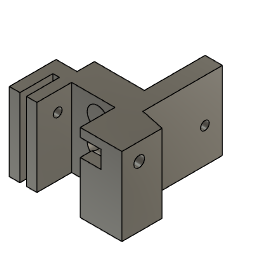
LeviDrzacZaALUProfilKojiDrziALUProfilSaGolmanom v4 (Autodesk Fusion 360 design; units mm, degrees)
Autodesk Fusion 360 part; units mm, degrees
note: some values were not read from the file. Set by a fixed rule: which sketch regions a step uses.
sketch "Sketch4" plane through (0, 0, 0) normal (0, 0, 1) x (1, 0, 0)
  line L0 (10, 0) -> (17, 0)
  line L1 (17, 0) -> (17, 20)
  line L2 (17, 20) -> (35, 20)
  line L3 (42, 27) -> (10, 27)
  line L4 (35, 20) -> (35, 0)
  line L5 (35, 0) -> (42, 0)
  line L6 (42, 0) -> (220, 0)
  line L7 (220, 0) -> (220, 27)
  line L8 (220, 27) -> (42, 27)
  line L9 (10, 27) -> (0, 27)
  line L10 (0, 0) -> (6.2, 0)
  line L11 (6.2, 0) -> (6.2, 19)
  line L12 (6.2, 19) -> (10, 19)
  line L13 (10, 19) -> (10, 0)
  line L14 (0.0791, 27) -> (0, 27)
  line L15 (0, 27) -> (0, 0)
  line L16 (0, 0) -> (0.0791, 0)
  line L17 (0.0791, 0) -> (0.0791, 27)
  dimension "d6" = 7
  dimension "d10" = 178
  dimension "d11" = 27
  dimension "d12" = 3.8
  constraint horizontal L0
  constraint vertical L1
  constraint horizontal L2
  constraint horizontal L3
  constraint vertical L4
  constraint horizontal L5
  constraint horizontal L6
  constraint vertical L7
  constraint horizontal L8
  constraint horizontal L9
  constraint horizontal L10
  constraint vertical L11
  constraint horizontal L12
  constraint vertical L13
  constraint horizontal L14
  constraint vertical L15
  constraint horizontal L16
  constraint vertical L17
  constraint coincident L10.start L15.end
  constraint coincident L9 L14.start
  constraint coincident L15 L10.start
  measures "d6" distance of L0.start L0.end
  measures "d10" distance of L5.end L6.end
  measures "d11" distance of L5.end L3.start
  measures "d12" distance of L0.start L10.end
extrude "Extrude1" add sketch "Sketch4" along normal blind 17 contours L0 L1 L2 L3 L4 L5 L6 L7 L8 L9 L10 L11 L12 L13 L17 makes body 1
sketch "Sketch5" plane through (0, 0, 0) normal (1, 0, 0) x (0, 1, 0)
  circle A0 centre (12, 9) radius 2.5
  dimension "d16" = 5
  measures "d16" diameter of A0
extrude "Extrude2" cut sketch "Sketch5" along normal blind 30 bodies 1
sketch "Sketch6" plane through (0, 0, 17) normal (0, 0, 1) x (-1, 0, 0)
  line L0 (-6.2, 0) -> (-6.2, -19)
  line L1 (-6.2, -19) -> (-10, -19)
  line L2 (-10, -19) -> (-10, 0)
  line L3 (-10, 0) -> (-17, 0)
  line L4 (-17, 0) -> (-17, -20)
  line L5 (-17, -20) -> (-35, -20)
  line L6 (-35, -20) -> (-35, 0)
  line L7 (-35, 0) -> (-220, 0)
  line L8 (-220, 0) -> (-220, -27)
  line L9 (-220, -27) -> (-0.0791, -27)
  line L10 (-0.0791, -27) -> (-0.0791, 0)
  line L11 (-0.0791, 0) -> (-6.2, 0)
  line L12 (-220, -27) -> (-42, -27)
  line L13 (-42, -27) -> (-42, -20)
  line L14 (-42, -20) -> (-220, -20)
  line L15 (-220, -20) -> (-220, -27)
  dimension "d19" = 178
  dimension "d20" = 7
  constraint horizontal L12
  constraint vertical L13
  constraint horizontal L14
  constraint vertical L15
  constraint coincident L8.end L9.start
  measures "d19" distance of L8.end L12.end
  measures "d20" distance of L8.end L14.end
extrude "Extrude3" cut sketch "Sketch6" against normal blind 60 contours L8 L9 L12 L13 L14 L15 bodies 1
sketch "Sketch7" plane through (0, 0, 17) normal (0, 0, 1) x (-1, 0, 0)
  line L0 (-42, -20) -> (-42, -27)
  line L1 (-42, -27) -> (-0.0791, -27)
  line L2 (-0.0791, -27) -> (-0.0791, 0)
  line L3 (-0.0791, 0) -> (-6.2, 0)
  line L4 (-6.2, 0) -> (-6.2, -19)
  line L5 (-6.2, -19) -> (-10, -19)
  line L6 (-10, -19) -> (-10, 0)
  line L7 (-10, 0) -> (-17, 0)
  line L8 (-17, 0) -> (-17, -20)
  line L9 (-17, -20) -> (-35, -20)
  line L10 (-35, -20) -> (-35, 0)
  line L11 (-35, 0) -> (-220, 0)
  line L12 (-220, 0) -> (-220, -20)
  line L13 (-220, -20) -> (-42, -20)
  line L14 (-42, -27) -> (-75, -20)
  constraint coincident L0.end L1.start
  constraint coincident L13 L14.end
extrude "Extrude4" add sketch "Sketch7" against normal blind 17 contours L0 L13 L14 bodies 1
sketch "Sketch8" plane through (0, 0, 17) normal (0, 0, 1) x (-1, 0, 0)
  line L0 (-42, -27) -> (-0.0791, -27)
  line L1 (-0.0791, -27) -> (-0.0791, 0)
  line L2 (-0.0791, 0) -> (-6.2, 0)
  line L3 (-6.2, 0) -> (-6.2, -19)
  line L4 (-6.2, -19) -> (-10, -19)
  line L5 (-10, -19) -> (-10, 0)
  line L6 (-10, 0) -> (-17, 0)
  line L7 (-17, 0) -> (-17, -20)
  line L8 (-17, -20) -> (-35, -20)
  line L9 (-35, -20) -> (-35, 0)
  line L10 (-35, 0) -> (-220, 0)
  line L11 (-220, 0) -> (-220, -20)
  line L12 (-220, -20) -> (-75, -20)
  line L13 (-75, -20) -> (-42, -27)
  line L14 (-17, -37) -> (-37, -37)
  line L15 (-17, -37) -> (-37, -37)
  line L16 (-37, -37) -> (-37, -85.9394)
  line L17 (-37, -85.9394) -> (-47, -85.9394)
  line L18 (-47, -85.9394) -> (-47, -25.9394)
  line L19 (-17, -37) -> (-17, -87)
  line L20 (-17, -87) -> (-7.161, -87)
  line L21 (-7.161, -87) -> (-7.161, -27)
  dimension "d26" = 20
  dimension "d27" = 10
  dimension "d28" = 60
  dimension "d29" = 60
  constraint perpendicular L14 L16
  constraint perpendicular L16 L17
  constraint coincident L13 L18.end
  constraint perpendicular L17 L18
  constraint perpendicular L14 L19
  constraint perpendicular L19 L20
  constraint coincident L0 L21.end
  constraint perpendicular L0 L21
  measures "d26" distance of L14.start L14.end
  measures "d27" distance of L16.end L17.end
  measures "d28" distance of L20.end L21.end
  measures "d29" distance of L17.end L18.end
extrude "Extrude5" add sketch "Sketch8" along normal blind 3 bodies 1
extrude "Extrude6" add 1 faces at (43.6667, 49.6263, 17) along direction (0, 0, -1) blind 17 on bodies 1 bodies 1
sketch "Sketch9" plane through (0, 20, 0) normal (0, -1, 0) x (1, 0, 0)
  line L0 (17, 0) -> (35, 0)
  line L1 (35, 0) -> (35, 20)
  line L2 (35, 20) -> (17, 20)
  line L3 (17, 20) -> (17, 0)
extrude "Extrude7" cut 1 faces at (35, 6.6667, 13.3333) along direction (1, 0, 0) blind 1 on bodies 1 bodies 1
extrude "Extrude8" cut 1 faces at (17, 3.176, 9.7909) along direction (-1, 0, 0) blind 1 on bodies 1 bodies 1
sketch "Sketch10" plane through (0, 20, 0) normal (0, -1, 0) x (1, 0, 0)
  arc A0 (26, 13.1) -> (22.9, 10) centre (26, 10) ccw
  circle A1 centre (26, 10) radius 3.1
  dimension "d40" = 6.2
  dimension "d41" = 6.2
  constraint concentric A0 A1
  measures "d40" diameter of A0
  measures "d41" diameter of A1
extrude "Extrude9" cut sketch "Sketch10" against normal blind 20 bodies 1
sketch "Sketch11" plane through (0, 20, 0) normal (0, -1, 0) x (1, 0, 0)
  circle A0 centre (26, 10) radius 6
  dimension "d44" = 12
  measures "d44" diameter of A0
extrude "Extrude10" cut sketch "Sketch11" against normal blind 5 bodies 1
sketch "Sketch12" plane through (47, 0, 0) normal (1, 0, 0) x (0, 1, 0)
  line L0 (85.9394, 0) -> (85.9394, 20)
  line L1 (85.9394, 20) -> (25.9394, 20)
  line L2 (25.9394, 20) -> (25.9394, 0)
  line L3 (25.9394, 0) -> (85.9394, 0)
  circle A0 centre (60, 10) radius 2.5
  dimension "d47" = 5
  measures "d47" diameter of A0
extrude "Extrude11" cut sketch "Sketch12" against normal blind 50 contours A0 bodies 1
sketch "Sketch13" plane through (0, 0, 20) normal (0, 0, 1) x (-1, 0, 0)
  line L0 (-16, -20) -> (-36, -20)
  line L1 (-36, -20) -> (-36, 0)
  line L2 (-36, 0) -> (-220, 0)
  line L3 (-220, 0) -> (-220, -20)
  line L4 (-220, -20) -> (-75, -20)
  line L5 (-75, -20) -> (-47, -25.9394)
  line L6 (-47, -25.9394) -> (-47, -85.9394)
  line L7 (-47, -85.9394) -> (-37, -85.9394)
  line L8 (-37, -85.9394) -> (-37, -37)
  line L9 (-37, -37) -> (-17, -37)
  line L10 (-17, -37) -> (-17, -87)
  line L11 (-17, -87) -> (-7.161, -87)
  line L12 (-7.161, -87) -> (-7.161, -27)
  line L13 (-7.161, -27) -> (-0.0791, -27)
  line L14 (-0.0791, -27) -> (-0.0791, 0)
  line L15 (-0.0791, 0) -> (-6.2, 0)
  line L16 (-6.2, 0) -> (-6.2, -19)
  line L17 (-6.2, -19) -> (-10, -19)
  line L18 (-10, -19) -> (-10, 0)
  line L19 (-10, 0) -> (-16, 0)
  line L20 (-16, 0) -> (-16, -20)
extrude "Extrude12" add 1 faces at (43.6667, 85.9394, 6.6667) along direction (0, 1, 0) blind 1.061 on bodies 1 bodies 1
sketch "Sketch14" plane through (0, 0, 20) normal (0, 0, 1) x (-1, 0, 0)
sketch "Sketch15" plane through (0, 37, 0) normal (0, 1, 0) x (-1, 0, 0)
  circle A0 centre (-26, 10) radius 3.1
  line L0 (-17, 0) -> (-17, 20)
  line L1 (-17, 20) -> (-37, 20)
  line L2 (-37, 20) -> (-37, 0)
  line L3 (-37, 0) -> (-17, 0)
  line L4 (-37, 10) -> (-27, 10)
  dimension "d52" = 10
  constraint midpoint L2 L4.start
  constraint perpendicular L2 L4
  measures "d52" distance of L4.start L4.end
extrude "Extrude13" add sketch "Sketch15" against normal blind 12 contours A0 bodies 1
sketch "Sketch16" plane through (0, 0, 20) normal (0, 0, 1) x (-1, 0, 0)
extrude "Extrude14" cut 1 faces at (17, 78.8333, 10) along direction (-1, 0, 0) blind 1 on bodies 1 bodies 1
sketch "Sketch17" plane through (0, 0, 20) normal (0, 0, 1) x (-1, 0, 0)
extrude "Extrude15" add 1 faces at (37, 78.8336, 10) along direction (-1, 0, 0) blind 1 on bodies 1 bodies 1
extrude "Extrude16" cut 1 faces at (47, 36.4596, 10) along direction (-1, 0, 0) blind 1 on bodies 1 bodies 1
sketch "Sketch18" plane through (0, 37, 0) normal (0, 1, 0) x (-1, 0, 0)
  line L0 (-36, 20) -> (-36, 0)
  line L1 (-36, 0) -> (-16, 0)
  line L2 (-16, 0) -> (-16, 20)
  line L3 (-16, 20) -> (-36, 20)
  circle A0 centre (-26, 10) radius 3.1
  dimension "d61" = 6.2
  measures "d61" diameter of A0
extrude "Extrude17" cut sketch "Sketch18" against normal blind 29 contours A0 bodies 1
sketch "Sketch19" plane through (0, 0, 20) normal (0, 0, 1) x (-1, 0, 0)
sketch "Sketch20" plane through (0, 0, 20) normal (0, 0, 1) x (-1, 0, 0)
  line L0 (-220, 0) -> (-60, 0)
  line L1 (-60, 0) -> (-60, -35)
  line L2 (-60, -35) -> (-237.965, -35)
  line L3 (-237.965, -35) -> (-237.965, 0)
  line L4 (-237.965, 0) -> (-220, 0)
  dimension "d64" = 160
  constraint horizontal L0
  constraint perpendicular L0 L1
  constraint perpendicular L1 L2
  constraint perpendicular L2 L3
  constraint perpendicular L3 L4
  measures "d64" distance of L0.start L0.end
extrude "Extrude18" cut sketch "Sketch20" against normal blind 40 bodies 1
sketch "Sketch21" plane through (60, 0, 0) normal (1, 0, 0) x (0, 1, 0)
  line L0 (23.1818, 0) -> (23.1818, 20)
  line L1 (23.1818, 20) -> (0, 20)
  line L2 (0, 20) -> (0, 0)
  line L3 (0, 0) -> (23.1818, 0)
  line L4 (0, 10) -> (10, 10)
  circle A0 centre (10, 10) radius 3.1
  dimension "d67" = 6.2
  constraint midpoint L2 L4.start
  constraint perpendicular L2 L4
  constraint coincident L4.end A0.centre
  measures "d67" diameter of A0
extrude "Extrude19" cut sketch "Sketch21" against normal blind 31 contours A0 bodies 1
sketch "Sketch22" plane through (36, 0, 0) normal (-1, 0, 0) x (0, -1, 0)
  circle A0 centre (-10, 10) radius 3.1
  line L0 (-20, 0) -> (0, 0)
  line L1 (0, 0) -> (0, 20)
  line L2 (0, 20) -> (-20, 20)
  line L3 (-20, 20) -> (-20, 0)
  circle A1 centre (-10, 10) radius 6
  dimension "d70" = 12
  constraint concentric A0 A1
  measures "d70" diameter of A1
extrude "Extrude20" cut sketch "Sketch22" against normal blind 6 contours A1 bodies 1
sketch "Sketch23" plane through (0, 0, 0) normal (0, -1, 0) x (1, 0, 0)
  line L0 (60, 0) -> (60, 20)
  line L1 (60, 20) -> (36, 20)
  line L2 (36, 20) -> (36, 0)
  line L3 (36, 0) -> (60, 0)
  line L4 (36, 15.0296) -> (48, 15.0296)
  line L5 (48, 15.0296) -> (48, 5)
  line L6 (48, 5) -> (36, 5)
  line L7 (36, 5) -> (36, 15.0296)
  dimension "d73" = 24
  dimension "d74" = 12
  constraint horizontal L4
  constraint vertical L5
  constraint horizontal L6
  constraint vertical L7
  constraint coincident L2 L4.start
  measures "d73" distance of L0.end L1.end
  measures "d74" distance of L4.start L4.end
extrude "Extrude21" cut sketch "Sketch23" against normal blind 10 contours L2 L4 L5 L6 L7 bodies 1
sketch "Sketch24" plane through (0, 0, 20) normal (0, 0, 1) x (-1, 0, 0)
sketch "Sketch25" plane through (0, 0, 0) normal (0, 0, -1) x (1, 0, 0)
  line L0 (60, -23.1818) -> (60, 0)
  line L1 (60, 0) -> (36, 0)
  line L2 (36, 0) -> (36, -20)
  line L3 (36, -20) -> (16, -20)
  line L4 (16, -20) -> (16, 0)
  line L5 (16, 0) -> (10, 0)
  line L6 (10, 0) -> (10, -19)
  line L7 (10, -19) -> (6.2, -19)
  line L8 (6.2, -19) -> (6.2, 0)
  line L9 (6.2, 0) -> (0.0791, 0)
  line L10 (0.0791, 0) -> (0.0791, -27)
  line L11 (0.0791, -27) -> (7.161, -27)
  line L12 (7.161, -27) -> (7.161, -87)
  line L13 (7.161, -87) -> (16, -87)
  line L14 (16, -87) -> (16, -37)
  line L15 (16, -37) -> (36, -37)
  line L16 (36, -37) -> (36, -87.0004)
  line L17 (36, -87.0004) -> (46, -87.0004)
  line L18 (46, -87.0004) -> (46, -25.9394)
  line L19 (46, -25.9394) -> (47, -25.9394)
  line L20 (47, -25.9394) -> (60, -23.1818)
  line L21 (46, -25.9394) -> (46, 0)
  line L22 (7.161, -27) -> (7.161, -19)
  constraint coincident L18.end L19.start
  constraint coincident L1 L21.end
  constraint perpendicular L1 L21
  constraint coincident L11.end L12.start
  constraint coincident L7 L22.end
  constraint perpendicular L7 L22
extrude "Extrude22" add sketch "Sketch25" along normal blind 15 contours L1 L2 L3 L4 L5 L6 L7 L12 L13 L14 L15 L16 L17 L18 L21 L22 bodies 1
sketch "Sketch26" plane through (0, 37, 0) normal (0, 1, 0) x (-1, 0, 0)
  circle A0 centre (-26, 10) radius 3.1
  line L0 (-36, 20) -> (-36, -15)
  line L1 (-36, -15) -> (-16, -15)
  line L2 (-16, -15) -> (-16, 20)
  line L3 (-16, 20) -> (-36, 20)
  circle A1 centre (-26, 10) radius 3.1
  constraint concentric A0 A1
extrude "Extrude23" add sketch "Sketch26" against normal blind 17 contours A0 A1 bodies 1
sketch "Sketch27" plane through (26, 20, 10) normal (0, -1, 0) x (1, 0, 0)
  circle A0 centre (0, 0) radius 5.984
  constraint coincident A0.centre origin
extrude "Extrude24" cut sketch "Sketch27" against normal blind 6 bodies 1
delete_face "DeleteFace1" 1 faces at (24.7178, 26, 11.1628) on bodies 1
sketch "Sketch28" plane through (26, 20, 10) normal (0, -1, 0) x (1, 0, 0)
sketch "Sketch29" plane through (0, 37, 0) normal (0, 1, 0) x (-1, 0, 0)
  line L0 (-36, 20) -> (-36, -15)
  line L1 (-36, -15) -> (-16, -15)
  line L2 (-16, -15) -> (-16, 20)
  line L3 (-16, 20) -> (-36, 20)
  circle A0 centre (-26, 10) radius 5.984
  circle A1 centre (-26, 10) radius 5.984
  constraint concentric A0 A1
extrude "Extrude25" add sketch "Sketch29" against normal blind 18 contours A0 A1 bodies 1
extrude "Extrude26" cut 1 faces at (24.2692, 19, 9.9802) along direction (0, 1, 0) blind 1 on bodies 1 bodies 1
sketch "Sketch30" plane through (46, 0, 0) normal (1, 0, 0) x (0, 1, 0)
  circle A0 centre (60, 10) radius 2.5
  line L0 (87.0004, 20) -> (25.9394, 20)
  line L1 (25.9394, 20) -> (25.9394, 0)
  line L2 (25.9394, 0) -> (0, 0)
  line L3 (0, 0) -> (0, -15)
  line L4 (0, -15) -> (87.0004, -15)
  line L5 (87.0004, -15) -> (87.0004, 20)
  circle A1 centre (60, 10) radius 2.5
  constraint concentric A0 A1
extrude "Extrude27" add sketch "Sketch30" against normal blind 10 contours A0 A1 bodies 1
sketch "Sketch31" plane through (7.161, 0, 0) normal (-1, 0, 0) x (0, -1, 0)
  circle A0 centre (-60, 10) radius 2.5
  line L0 (-27, 0) -> (-27, 20)
  line L1 (-27, 20) -> (-87, 20)
  line L2 (-87, 20) -> (-87, -15)
  line L3 (-87, -15) -> (-19, -15)
  line L4 (-19, -15) -> (-19, 0)
  line L5 (-19, 0) -> (-27, 0)
extrude "Extrude28" add sketch "Sketch31" against normal blind 10 contours A0 bodies 1
extrude "Extrude29" cut 1 faces at (17.161, 60.3667, 10.0553) along direction (-1, 0, 0) blind 1 on bodies 1 bodies 1
sketch "Sketch32" plane through (16, 0, 0) normal (1, 0, 0) x (0, 1, 0)
  circle A0 centre (60, 10) radius 2.5
  line L0 (87, -15) -> (87, 20)
  line L1 (87, 20) -> (37, 20)
  line L2 (37, 20) -> (37, -15)
  line L3 (37, -15) -> (87, -15)
  circle A1 centre (60, 10) radius 6.7082
  constraint concentric A0 A1
extrude "Extrude30" cut sketch "Sketch32" against normal blind 10 contours A1 bodies 1 makes body 2 at (46, 66.6467, 1.6667)
extrude "Extrude31" cut 1 faces at (16.161, 60.3667, 10.0553) along direction (-1, 0, 0) blind 10 on bodies 1 bodies 1
sketch "Sketch33" plane through (0, 0, 0) normal (0, 1, 0) x (1, 0, 0)
  circle A0 centre (3577.0001, -10) radius 500
sketch "Sketch34" plane through (7.161, 0, 0) normal (-1, 0, 0) x (0, -1, 0)
  line L0 (-27, 0) -> (-27, 20)
  line L1 (-27, 20) -> (-87, 20)
  line L2 (-87, 20) -> (-87, -15)
  line L3 (-87, -15) -> (-19, -15)
  line L4 (-19, -15) -> (-19, 0)
  line L5 (-19, 0) -> (-27, 0)
  circle A0 centre (-60, 10) radius 6.7082
  circle A1 centre (-60, 10) radius 6.7082
  constraint concentric A0 A1
extrude "Extrude32" add sketch "Sketch34" against normal blind 10 contours A0 A1 bodies 1 2
extrude "Extrude33" cut 1 faces at (17.161, 57.9973, 13.1138) along direction (-1, 0, 0) blind 1 on bodies 1 bodies 1
sketch "Sketch35" plane through (0, 0, 20) normal (0, 0, 1) x (-1, 0, 0)
  line L0 (-36, -37) -> (-46, -37)
  constraint horizontal L0
sketch "Sketch36" plane through (46, 0, 0) normal (1, 0, 0) x (0, 1, 0)
  line L0 (87.0004, 20) -> (25.9394, 20)
  line L1 (25.9394, 20) -> (25.9394, 0)
  line L2 (25.9394, 0) -> (0, 0)
  line L3 (0, 0) -> (0, -15)
  line L4 (0, -15) -> (87.0004, -15)
  line L5 (87.0004, -15) -> (87.0004, 20)
  line L6 (36.8806, 20) -> (36.8806, -6.3582)
  line L7 (36.8806, -6.3582) -> (36.8806, -15)
  line L8 (36.8806, -15) -> (36.8806, -5)
  line L9 (36.8806, -5) -> (61.8806, -5)
  circle A0 centre (61.8806, -5) radius 2.5
  dimension "d101" = 10
  dimension "d102" = 25
  dimension "d103" = 5
  constraint coincident L0 L6.start
  constraint perpendicular L0 L6
  constraint perpendicular L0 L7
  constraint perpendicular L4 L8
  constraint perpendicular L8 L9
  constraint coincident L9.end A0.centre
  measures "d101" distance of L7.end L8.end
  measures "d102" distance of L8.end L9.end
  measures "d103" diameter of A0
extrude "Extrude34" cut sketch "Sketch36" against normal blind 10 contours A0 bodies 1
sketch "Sketch37" plane through (0, 0, -15) normal (0, 0, -1) x (1, 0, 0)
  line L0 (7.161, -87) -> (16, -87)
  line L1 (16, -87) -> (16, -37)
  line L2 (16, -37) -> (36, -37)
  line L3 (36, -37) -> (36, -87.0004)
  line L4 (36, -87.0004) -> (46, -87.0004)
  line L5 (46, -87.0004) -> (46, 0)
  line L6 (46, 0) -> (36, 0)
  line L7 (36, 0) -> (36, -20)
  line L8 (36, -20) -> (16, -20)
  line L9 (16, -20) -> (16, 0)
  line L10 (16, 0) -> (10, 0)
  line L11 (10, 0) -> (10, -19)
  line L12 (10, -19) -> (7.161, -19)
  line L13 (7.161, -19) -> (7.161, -87)
sketch "Sketch38" plane through (7.161, 0, 0) normal (-1, 0, 0) x (0, -1, 0)
  line L0 (-27, 0) -> (-27, 20)
  line L1 (-27, 20) -> (-87, 20)
  line L2 (-87, 20) -> (-87, -15)
  line L3 (-87, -15) -> (-19, -15)
  line L4 (-19, -15) -> (-19, 0)
  line L5 (-19, 0) -> (-27, 0)
  line L6 (-36.9806, -15) -> (-36.9806, 12.6008)
  line L7 (-36.9806, 20) -> (-36.9806, 10)
  line L8 (-36.9806, -15) -> (-36.9806, -5)
  line L9 (-36.9806, -5) -> (-61.9806, -5)
  circle A0 centre (-61.9806, -5) radius 2.5
  dimension "d106" = 10
  dimension "d107" = 10
  dimension "d108" = 25
  dimension "d109" = 5
  constraint coincident L3 L6.start
  constraint perpendicular L3 L6
  constraint coincident L1 L7.start
  constraint perpendicular L1 L7
  constraint perpendicular L3 L8
  constraint perpendicular L6 L9
  constraint coincident L9.end A0.centre
  measures "d106" distance of L7.start L7.end
  measures "d107" distance of L6.start L8.end
  measures "d108" distance of L8.end L9.end
  measures "d109" diameter of A0
extrude "Extrude35" cut sketch "Sketch38" against normal blind 10 contours A0 bodies 1
sketch "Sketch39" plane through (0, 20, 0) normal (0, -1, 0) x (1, 0, 0)
  circle A0 centre (26, 10) radius 6
  line L0 (36, -15) -> (36, 20)
  line L1 (36, 20) -> (16, 20)
  line L2 (16, 20) -> (16, -15)
  line L3 (16, -15) -> (36, -15)
  line L4 (25, -15) -> (25, -5)
  circle A1 centre (25, -5) radius 3.1
  dimension "d112" = 10
  dimension "d113" = 6.2
  constraint coincident L3 L4.start
  constraint perpendicular L3 L4
  constraint coincident L4.end A1.centre
  measures "d112" distance of L4.start L4.end
  measures "d113" diameter of A1
extrude "Extrude36" cut sketch "Sketch39" against normal blind 20 contours A1 bodies 1
sketch "Sketch40" plane through (0, 20, 0) normal (0, -1, 0) x (1, 0, 0)
  circle A0 centre (25, -5) radius 3.1
  circle A1 centre (26, 10) radius 6
  line L0 (36, -15) -> (36, 20)
  line L1 (36, 20) -> (16, 20)
  line L2 (16, 20) -> (16, -15)
  line L3 (16, -15) -> (36, -15)
  circle A2 centre (25, -5) radius 6
  dimension "d116" = 12
  constraint concentric A0 A2
  measures "d116" diameter of A2
extrude "Extrude37" cut sketch "Sketch40" against normal blind 6 contours A2 bodies 1
sketch "Sketch41" plane through (0, -17.4661, 0) normal (0, -1, 0) x (1, 0, 0)
  line L0 (173.7484, 48.8339) -> (173.7484, 63.8339)
  line L1 (173.7484, 63.8339) -> (153.7484, 63.8339)
  line L2 (153.7484, 63.8339) -> (153.7484, 48.8339)
  line L3 (153.7484, 63.8339) -> (163.7484, 63.8339)
  line L4 (163.7484, 63.8339) -> (163.7484, 53.8339)
  circle A0 centre (163.7484, 53.8339) radius 3.1
  line L5 (153.7484, 48.8339) -> (173.7484, 48.8339)
  dimension "d123" = 10
  dimension "d124" = 10
  dimension "d125" = 6.2
  constraint coincident L1.end L2.start
  constraint perpendicular L2 L3
  constraint perpendicular L1 L4
  constraint coincident L4.end A0.centre
  measures "d123" distance of L1.end L3.end
  measures "d124" distance of L3.end L4.end
  measures "d125" diameter of A0
sketch "Sketch42" plane through (0, -17.4661, 0) normal (0, -1, 0) x (1, 0, 0)
  circle A0 centre (163.7484, 53.8339) radius 3.1
  line L0 (173.7484, 48.8339) -> (173.7484, 63.8339)
  line L1 (173.7484, 63.8339) -> (153.7484, 63.8339)
  line L2 (153.7484, 63.8339) -> (153.7484, 48.8339)
  circle A1 centre (163.7484, 53.8339) radius 6
  line L3 (153.7484, 48.8339) -> (173.7484, 48.8339)
  dimension "d128" = 12
  constraint concentric A0 A1
  measures "d128" diameter of A1
extrude "Extrude42" cut 1 faces at (29.9995, 26, -5.4521) along direction (0, 1, 0) blind 20 on bodies 1 bodies 1
sketch "Sketch43" plane through (0, 20, 0) normal (0, -1, 0) x (1, 0, 0)
  circle A0 centre (25, -5) radius 6
  circle A1 centre (26, 10) radius 6
  line L0 (36, -15) -> (36, 20)
  line L1 (36, 20) -> (16, 20)
  line L2 (16, 20) -> (16, -15)
  line L3 (16, -15) -> (36, -15)
  circle A2 centre (25, -5) radius 6
  dimension "d133" = 12
  constraint concentric A0 A2
  measures "d133" diameter of A2
extrude "Extrude43" add sketch "Sketch43" against normal blind 20 contours A0 A2 bodies 1
sketch "Sketch44" plane through (0, 20, 0) normal (0, -1, 0) x (1, 0, 0)
  circle A0 centre (26, 10) radius 6
  line L0 (36, -15) -> (36, 20)
  line L1 (36, 20) -> (16, 20)
  line L2 (16, 20) -> (16, -15)
  line L3 (16, -15) -> (36, -15)
  line L4 (16, -15) -> (26, -15)
  line L5 (26, -15) -> (26, -5)
  circle A1 centre (26, -5) radius 3.1
  dimension "d136" = 10
  dimension "d137" = 10
  dimension "d138" = 6.2
  constraint coincident L2.end L3.start
  constraint perpendicular L2 L4
  constraint perpendicular L4 L5
  constraint coincident L5.end A1.centre
  measures "d136" distance of L2.end L4.end
  measures "d137" distance of L4.end L5.end
  measures "d138" diameter of A1
extrude "Extrude44" cut sketch "Sketch44" against normal blind 20 contours A1 bodies 1
sketch "Sketch45" plane through (0, 20, 0) normal (0, -1, 0) x (1, 0, 0)
  circle A0 centre (26, -5) radius 3.1
  circle A1 centre (26, 10) radius 6
  line L0 (36, -15) -> (36, 20)
  line L1 (36, 20) -> (16, 20)
  line L2 (16, 20) -> (16, -15)
  line L3 (16, -15) -> (36, -15)
  circle A2 centre (26, -5) radius 6
  dimension "d141" = 12
  constraint concentric A0 A2
  measures "d141" diameter of A2
extrude "Extrude45" cut sketch "Sketch45" against normal blind 6 contours A2 bodies 1
sketch "Sketch46" plane through (0, 0, 63.8339) normal (0, 0, 1) x (-1, 0, 0)
  line L0 (-197.7484, 37.4661) -> (-197.7484, 14.2843)
  line L1 (-197.7484, 14.2843) -> (-184.7484, 11.5267)
  line L2 (-184.7484, 11.5267) -> (-183.7484, 11.5267)
  line L3 (-183.7484, 11.5267) -> (-183.7484, -49.5343)
  line L4 (-183.7484, -49.5343) -> (-173.7484, -49.5343)
  line L5 (-173.7484, -49.5343) -> (-173.7484, 0.4661)
  line L6 (-173.7484, 0.4661) -> (-153.7484, 0.4661)
  line L7 (-153.7484, 0.4661) -> (-153.7484, -49.5339)
  line L8 (-153.7484, -49.5339) -> (-144.9094, -49.5339)
  line L9 (-144.9094, -49.5339) -> (-144.9094, 10.4661)
  line L10 (-144.9094, 10.4661) -> (-137.8275, 10.4661)
  line L11 (-137.8275, 10.4661) -> (-137.8275, 37.4661)
  line L12 (-137.8275, 37.4661) -> (-143.9484, 37.4661)
  line L13 (-143.9484, 37.4661) -> (-143.9484, 18.4661)
  line L14 (-143.9484, 18.4661) -> (-147.7484, 18.4661)
  line L15 (-147.7484, 18.4661) -> (-147.7484, 37.4661)
  line L16 (-147.7484, 37.4661) -> (-153.7484, 37.4661)
  line L17 (-153.7484, 37.4661) -> (-153.7484, 17.4661)
  line L18 (-153.7484, 17.4661) -> (-173.7484, 17.4661)
  line L19 (-173.7484, 17.4661) -> (-173.7484, 37.4661)
  line L20 (-173.7484, 37.4661) -> (-197.7484, 37.4661)
  line L21 (-173.7484, 0.4661) -> (-183.7484, 0.4661)
  line L22 (-183.7484, 0.4661) -> (-144.9094, 0.4661)
  constraint coincident L5.end L6.start
  constraint coincident L3 L21.end
  constraint perpendicular L3 L21
  constraint coincident L9 L22.end
  constraint perpendicular L9 L22
sketch "Sketch47" plane through (183.7484, 0, 0) normal (1, 0, 0) x (0, 1, 0)
  line L0 (49.5343, 48.8339) -> (49.5343, 63.8339)
  line L1 (49.5343, 63.8339) -> (-11.5267, 63.8339)
  line L2 (-11.5267, 63.8339) -> (-11.5267, 48.8339)
  line L3 (-0.4671, 63.8339) -> (-0.4671, 28.8339)
  line L4 (-0.4671, 63.8339) -> (-0.4671, 53.8339)
  line L5 (-0.4671, 53.8339) -> (24.5329, 53.8339)
  circle A0 centre (24.5329, 53.8339) radius 2.5
  line L6 (-11.5267, 48.8339) -> (49.5343, 48.8339)
  dimension "d144" = 10
  dimension "d145" = 25
  dimension "d146" = 5
  constraint coincident L1 L3.start
  constraint perpendicular L1 L4
  constraint perpendicular L3 L5
  constraint coincident L5.end A0.centre
  measures "d144" distance of L3.start L4.end
  measures "d145" distance of L4.end L5.end
  measures "d146" diameter of A0
sketch "Sketch48" plane through (144.9094, 0, 0) normal (-1, 0, 0) x (0, -1, 0)
  line L0 (10.4661, 48.8339) -> (10.4661, 63.8339)
  line L1 (10.4661, 63.8339) -> (-49.5339, 63.8339)
  line L2 (-49.5339, 63.8339) -> (-49.5339, 48.8339)
  line L3 (0.3737, 63.8339) -> (0.3737, 53.8339)
  line L4 (0.3737, 53.8339) -> (-24.6263, 53.8339)
  circle A0 centre (-24.6263, 53.8339) radius 2.5
  line L5 (-49.5339, 48.8339) -> (10.4661, 48.8339)
  dimension "d149" = 10
  dimension "d150" = 25
  dimension "d151" = 5
  constraint coincident L1 L3.start
  constraint perpendicular L1 L3
  constraint perpendicular L3 L4
  constraint coincident L4.end A0.centre
  measures "d149" distance of L3.start L3.end
  measures "d150" distance of L3.end L4.end
  measures "d151" diameter of A0
extrude "Extrude48" add 1 faces at (51, 16.3737, 0) along direction (0, 0, -1) blind 15 on bodies 1 bodies 1
extrude "Extrude49" add 1 faces at (2.1194, 15.3333, 0) along direction (0, 0, -1) blind 15 on bodies 1 bodies 1
extrude "Extrude50" cut 1 faces at (20.4227, 40, -6.0416) along direction (0, -1, 0) blind 3 on bodies 1 bodies 1
move_body "Move4" bodies 1 to x (1, 0, 0) y (0, 1, 0) z (0, 0, 1) at (0, 0, 15)
sketch "Sketch49" plane through (0, 0, -15) normal (0, 0, -1) x (1, 0, 0)
sketch "Sketch50" plane through (0, 0, -15) normal (0, 0, -1) x (1, 0, 0)
sketch "Sketch51" plane through (0, 0, 0) normal (0, 0, -1) x (1, 0, 0)
  line L0 (7.161, -87) -> (16, -87)
  line L1 (16, -87) -> (16, -37)
  line L2 (16, -37) -> (36, -37)
  line L3 (36, -37) -> (36, -87.0004)
  line L4 (36, -87.0004) -> (46, -87.0004)
  line L5 (46, -87.0004) -> (46, -25.9394)
  line L6 (46, -25.9394) -> (47, -25.9394)
  line L7 (47, -25.9394) -> (60, -23.1818)
  line L8 (60, -23.1818) -> (60, 0)
  line L9 (60, 0) -> (36, 0)
  line L10 (36, 0) -> (36, -20)
  line L11 (36, -20) -> (16, -20)
  line L12 (16, -20) -> (16, 0)
  line L13 (16, 0) -> (10, 0)
  line L14 (10, 0) -> (10, -19)
  line L15 (10, -19) -> (6.2, -19)
  line L16 (6.2, -19) -> (6.2, 0)
  line L17 (6.2, 0) -> (0.0791, 0)
  line L18 (0.0791, 0) -> (0.0791, -27)
  line L19 (0.0791, -27) -> (7.161, -27)
  line L20 (7.161, -27) -> (7.161, -87)
  line L21 (36, -37) -> (7.161, -37)
  constraint coincident L2.end L3.start
  constraint coincident L20 L21.end
  constraint perpendicular L20 L21
sketch "Sketch52" plane through (0, 37, 0) normal (0, 1, 0) x (-1, 0, 0)
  circle A0 centre (-26, 10) radius 3.1
  line L0 (-36, 35) -> (-36, 0)
  line L1 (-36, 0) -> (-16, 0)
  line L2 (-16, 35) -> (-36, 35)
  line L3 (-16, 0) -> (-16, 35)
extrude "Extrude53" add 1 faces at (44, 6.6667, 0) along direction (0, 0, -1) blind 10 on bodies 1 bodies 1
sketch "Sketch53" plane through (0, 37, 0) normal (0, 1, 0) x (-1, 0, 0)
  circle A0 centre (-26, 10) radius 3.1
  line L0 (-36, 35) -> (-36, -10)
  line L1 (-36, -10) -> (-16, -10)
  line L2 (-16, 35) -> (-36, 35)
  line L3 (-36, -10) -> (-36, 0)
  line L4 (-36, 0) -> (-7.161, 0)
  line L5 (-16, -10) -> (-16, 35)
  dimension "d166" = 10
  constraint coincident L0.end L1.start
  constraint perpendicular L1 L3
  measures "d166" distance of L0.end L3.end
extrude "Extrude54" add sketch "Sketch53" along normal blind 50 contours L0 L1 L3 L4 L5 bodies 1
sketch "Sketch54" plane through (0, 0, -10) normal (0, 0, -1) x (1, 0, 0)
  line L0 (7.161, -27) -> (7.161, -87)
  line L1 (7.161, -87) -> (36, -87)
  line L2 (36, -87) -> (36, -87.0004)
  line L3 (36, -87.0004) -> (46, -87.0004)
  line L4 (46, -87.0004) -> (46, -25.9394)
  line L5 (46, -25.9394) -> (47, -25.9394)
  line L6 (47, -25.9394) -> (60, -23.1818)
  line L7 (60, -23.1818) -> (60, 0)
  line L8 (60, 0) -> (36, 0)
  line L9 (36, 0) -> (36, -20)
  line L10 (36, -20) -> (16, -20)
  line L11 (16, -20) -> (16, 0)
  line L12 (16, 0) -> (10, 0)
  line L13 (10, 0) -> (10, -19)
  line L14 (10, -19) -> (6.2, -19)
  line L15 (6.2, -19) -> (6.2, 0)
  line L16 (6.2, 0) -> (0.0791, 0)
  line L17 (0.0791, 0) -> (0.0791, -27)
  line L18 (0.0791, -27) -> (7.161, -27)
  line L19 (36, -37) -> (16, -37)
  line L20 (16, -37) -> (26, -37)
  line L21 (26, -37) -> (26, -62)
  circle A0 centre (26, -62) radius 2.5
  dimension "d169" = 25
  dimension "d170" = 5
  constraint horizontal L19
  constraint midpoint L19 L20.end
  constraint perpendicular L19 L21
  constraint coincident L21.end A0.centre
  measures "d169" distance of L20.end L21.end
  measures "d170" diameter of A0
extrude "Extrude55" cut sketch "Sketch54" against normal blind 11 contours A0 bodies 1
sketch "Sketch55" plane through (0, 0, 0) normal (0, 0, 1) x (-1, 0, 0)
  circle A0 centre (-26, -62) radius 2.5
  line L0 (-16, -37) -> (-36, -37)
  line L1 (-36, -37) -> (-36, -87)
  line L2 (-36, -87) -> (-16, -87)
  line L3 (-16, -87) -> (-16, -37)
sketch "Sketch56" plane through (36, 0, 0) normal (-1, 0, 0) x (0, -1, 0)
  line L0 (-87, 0) -> (-37, 0)
  line L1 (-37, 0) -> (-37, 35)
  line L2 (-37, 35) -> (-87.0004, 35)
  line L3 (-87.0004, 35) -> (-87.0004, -10)
  line L4 (-87.0004, -10) -> (-87, -10)
  line L5 (-87, -10) -> (-87, 0)
  circle A0 centre (-61.8806, 10) radius 2.5
move_body "Move5" bodies 1 to x (1, 0, 0) y (0, 1, 0) z (0, 0, 1) at (0, 0, 10)
sketch "Sketch57" plane through (0, 87, 0) normal (0, 1, 0) x (-1, 0, 0)
  line L0 (-16, 45) -> (-16, 10)
  line L1 (-16, 10) -> (-36, 10)
  line L2 (-36, 10) -> (-36, 0)
  line L3 (-36, 0) -> (-7.161, 0)
  line L4 (-7.161, 0) -> (-7.161, 45)
  line L5 (-7.161, 45) -> (-16, 45)
  line L6 (-16, 10) -> (-7.161, 10)
  constraint coincident L0.end L1.start
  constraint coincident L4 L6.end
  constraint perpendicular L4 L6
sketch "Sketch58" plane through (0, 87, 0) normal (0, 1, 0) x (-1, 0, 0)
  line L0 (-16, 45) -> (-16, 10)
  line L1 (-16, 10) -> (-36, 10)
  line L2 (-36, 10) -> (-36, 0)
  line L3 (-36, 0) -> (-7.161, 0)
  line L4 (-7.161, 0) -> (-7.161, 45)
  line L5 (-7.161, 45) -> (-16, 45)
  line L6 (-16, 10) -> (-7.161, 10)
  constraint coincident L0.end L1.start
  constraint coincident L4 L6.end
  constraint perpendicular L4 L6
extrude "Extrude56" cut 1 faces at (16.161, 57.9973, 38.1138) along direction (-1, 0, 0) blind 30 on bodies 1 bodies 1
sketch "Sketch59" plane through (0, 87, 0) normal (0, 1, 0) x (-1, 0, 0)
  line L0 (-16, 45) -> (-16, 10)
  line L1 (-16, 10) -> (-36, 10)
  line L2 (-36, 10) -> (-36, 0)
  line L3 (-36, 0) -> (-7.161, 0)
  line L4 (-7.161, 0) -> (-7.161, 45)
  line L5 (-7.161, 45) -> (-16, 45)
  line L6 (-16, 45) -> (-7.161, 45)
  line L7 (-7.161, 45) -> (-7.161, 9.8705)
  line L8 (-7.161, 9.8705) -> (-16, 9.8705)
  line L9 (-16, 9.8705) -> (-16, 45)
  constraint horizontal L6
  constraint vertical L7
  constraint horizontal L8
  constraint vertical L9
  constraint coincident L4 L7.end
  constraint coincident L0.start L5.end
extrude "Extrude57" cut sketch "Sketch58" against normal blind 50 contours L0 L4 L5 L6 bodies 1
extrude "Extrude58" add 1 faces at (0.0791, 13.0623, 10.5023) along direction (-1, 0, 0) blind 5 on bodies 1 bodies 1
extrude "Extrude59" cut 1 faces at (6.2, 10.2711, 10.5023) along direction (-1, 0, 0) blind 5 on bodies 1 bodies 1
extrude "Extrude60" add 1 faces at (10, 10.2711, 10.5023) along direction (-1, 0, 0) blind 5 on bodies 1 bodies 1
extrude "Extrude61" cut 1 faces at (16, 10.6044, 10.5023) along direction (-1, 0, 0) blind 5 on bodies 1 bodies 1
sketch "Sketch60" plane through (0, 0, 45) normal (0, 0, 1) x (-1, 0, 0)
  line L0 (-11, -20) -> (-36, -20)
  line L1 (-36, -20) -> (-36, 0)
  line L2 (-36, 0) -> (-60, 0)
  line L3 (-60, 0) -> (-60, -23.1818)
  line L4 (-60, -23.1818) -> (-47, -25.9394)
  line L5 (-47, -25.9394) -> (-46, -25.9394)
  line L6 (-46, -25.9394) -> (-46, -87.0004)
  line L7 (-46, -87.0004) -> (-36, -87.0004)
  line L8 (-36, -87.0004) -> (-36, -37)
  line L9 (-36, -37) -> (-7.161, -37)
  line L10 (-7.161, -37) -> (-7.161, -27)
  line L11 (-7.161, -27) -> (4.9209, -27)
  line L12 (4.9209, -27) -> (4.9209, 0)
  line L13 (4.9209, 0) -> (-1.2, 0)
  line L14 (-1.2, 0) -> (-1.2, -19)
  line L15 (-1.2, -19) -> (-5, -19)
  line L16 (-5, -19) -> (-5, 0)
  line L17 (-5, 0) -> (-11, 0)
  line L18 (-11, 0) -> (-11, -20)
extrude "Extrude62" cut 1 faces at (42.6667, 87.0004, 15) along direction (0, -1, 0) blind 10 on bodies 1 bodies 1
extrude "Extrude63" cut 1 faces at (16.774, 87, 3.3333) along direction (0, -1, 0) blind 10 on bodies 1 bodies 1
sketch "Sketch61" plane through (0, 0, 45) normal (0, 0, 1) x (-1, 0, 0)
  line L0 (-46, -77.0004) -> (-36, -77.0004)
  line L1 (-36, -77.0004) -> (-36, -37)
  line L2 (-36, -37) -> (-7.161, -37)
  line L3 (-7.161, -37) -> (-7.161, -27)
  line L4 (-7.161, -27) -> (4.9209, -27)
  line L5 (4.9209, -27) -> (4.9209, 0)
  line L6 (4.9209, 0) -> (-1.2, 0)
  line L7 (-1.2, 0) -> (-1.2, -19)
  line L8 (-1.2, -19) -> (-5, -19)
  line L9 (-5, -19) -> (-5, 0)
  line L10 (-5, 0) -> (-11, 0)
  line L11 (-11, 0) -> (-11, -20)
  line L12 (-11, -20) -> (-36, -20)
  line L13 (-36, -20) -> (-36, 0)
  line L14 (-36, 0) -> (-60, 0)
  line L15 (-60, 0) -> (-60, -23.1818)
  line L16 (-60, -23.1818) -> (-47, -25.9394)
  line L17 (-47, -25.9394) -> (-46, -25.9394)
  line L18 (-46, -25.9394) -> (-46, -77.0004)
extrude "Extrude64" cut 1 faces at (42.6667, 77.0004, 15) along direction (0, -1, 0) blind 5 on bodies 1 bodies 1
extrude "Extrude65" cut 1 faces at (16.774, 77, 3.3333) along direction (0, -1, 0) blind 5 on bodies 1 bodies 1
